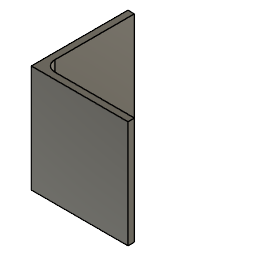
L-90×90×6 (Autodesk Fusion 360 design; units mm, degrees)
Autodesk Fusion 360 part; units mm, degrees
note: some values were not read from the file. Set by a fixed rule: which sketch regions a step uses.
sketch "スケッチ1" plane through (0, 0, 0) normal (0, 0, 1) x (1, 0, 0)
  line L0 (90, 6) -> (16, 6)
  line L1 (0, 0) -> (90, 0)
  line L2 (0, 90) -> (0, 0)
  line L3 (6, 16) -> (6, 90)
  arc A0 (6, 16) -> (16, 6) centre (16, 16) ccw
  line L4 (6, 90) -> (0, 90)
  line L5 (90, 0) -> (90, 6)
extrude "押し出し1" add sketch "スケッチ1" along normal blind 100
